Autodesk Fusion 360 part; units mm, degrees
(part 2 of 5)
  spline S301 degree 3 poles (-67.6031, -107.6158) (-67.9091, -107.753) (-68.2046, -107.8902) (-68.2574, -107.9113) knots 0 0 0 0 1 1 1 1
  spline S302 degree 3 poles (-68.2574, -107.9113) (-68.3629, -107.964) (-68.0041, -107.4364) (-67.5926, -106.9088) knots 0 0 0 0 1 1 1 1
  spline S303 degree 3 poles (-67.5926, -106.9088) (-67.276, -106.5289) (-67.1599, -106.4867) (-67.1599, -106.74) knots 0 0 0 0 1 1 1 1
  spline S304 degree 3 poles (-43.6395, -107.6791) (-43.4495, -107.9324) (-43.3229, -108.1434) (-43.344, -108.1434) knots 0 0 0 0 1 1 1 1
  spline S305 degree 3 poles (-43.344, -108.1434) (-43.3757, -108.1434) (-43.6078, -108.0273) (-43.8505, -107.8796) knots 0 0 0 0 1 1 1 1
  spline S306 degree 3 poles (-43.8505, -107.8796) (-44.1038, -107.7319) (-44.4098, -107.6158) (-44.5258, -107.6158) knots 0 0 0 0 1 1 1 1
  spline S307 degree 3 poles (-44.5258, -107.6158) (-44.9901, -107.6158) (-45.064, -107.2676) (-44.6947, -106.8772) knots 0 0 0 0 1 1 1 1
  spline S308 degree 3 poles (-44.6947, -106.8772) (-44.5364, -106.7083) (-44.5047, -106.7189) (-44.2515, -106.951) knots 0 0 0 0 1 1 1 1
  spline S309 degree 3 poles (-44.2515, -106.951) (-44.0932, -107.0988) (-43.8189, -107.4153) (-43.6395, -107.6791) knots 0 0 0 0 1 1 1 1
  spline S310 degree 3 poles (-45.3172, -106.9827) (-45.0323, -106.9827) (-45.0007, -107.0038) (-45.064, -107.2465) knots 0 0 0 0 1 1 1 1
  spline S311 degree 3 poles (-45.064, -107.2465) (-45.1062, -107.4364) (-45.0745, -107.5314) (-44.9585, -107.5736) knots 0 0 0 0 1 1 1 1
  spline S312 degree 3 poles (-44.9585, -107.5736) (-44.8424, -107.6158) (-44.8213, -107.6791) (-44.8952, -107.8057) knots 0 0 0 0 1 1 1 1
  spline S313 degree 3 poles (-44.8952, -107.8057) (-45.1695, -108.2911) (-45.1695, -108.2911) (-45.676, -107.9218) knots 0 0 0 0 1 1 1 1
  spline S314 degree 3 poles (-45.676, -107.9218) (-45.982, -107.7108) (-46.1508, -107.5208) (-46.1086, -107.4259) knots 0 0 0 0 1 1 1 1
  spline S315 degree 3 poles (-46.1086, -107.4259) (-46.077, -107.352) (-46.0559, -107.1621) (-46.0559, -107.0249) knots 0 0 0 0 1 1 1 1
  spline S316 degree 3 poles (-46.0559, -107.0249) (-46.0559, -106.8033) (-46.0242, -106.7822) (-45.8554, -106.8772) knots 0 0 0 0 1 1 1 1
  spline S317 degree 3 poles (-45.8554, -106.8772) (-45.7393, -106.9299) (-45.4966, -106.9827) (-45.3172, -106.9827) knots 0 0 0 0 1 1 1 1
  spline S318 degree 3 poles (-43.5234, -108.2173) (-42.2677, -108.9454) (-41.0542, -110.1166) (-40.5161, -111.1296) knots 0 0 0 0 1 1 1 1
  line L66 (-40.5161, -111.1296) -> (-40.2206, -111.6783)
  line L67 (-40.2206, -111.6783) -> (-40.6955, -111.2352)
  spline S319 degree 3 poles (-40.6955, -111.2352) (-41.4341, -110.5704) (-42.6792, -110.0006) (-43.6817, -109.8739) knots 0 0 0 0 1 1 1 1
  spline S320 degree 3 poles (-43.6817, -109.8739) (-44.2304, -109.8001) (-44.3042, -109.9161) (-43.7661, -110.0006) knots 0 0 0 0 1 1 1 1
  spline S321 degree 3 poles (-43.7661, -110.0006) (-42.8164, -110.1483) (-42.5632, -110.3804) (-42.1516, -111.4884) knots 0 0 0 0 1 1 1 1
  spline S322 degree 3 poles (-42.1516, -111.4884) (-41.8984, -112.1743) (-41.7295, -112.8918) (-41.8245, -112.8813) knots 0 0 0 0 1 1 1 1
  spline S323 degree 3 poles (-41.8245, -112.8813) (-41.8562, -112.8813) (-42.1516, -112.5647) (-42.4682, -112.1848) knots 0 0 0 0 1 1 1 1
  spline S324 degree 3 poles (-42.4682, -112.1848) (-43.0591, -111.4779) (-44.5153, -110.1905) (-45.2328, -109.7473) knots 0 0 0 0 1 1 1 1
  spline S325 degree 3 poles (-45.2328, -109.7473) (-45.581, -109.5363) (-45.6127, -109.473) (-45.5072, -109.3041) knots 0 0 0 0 1 1 1 1
  spline S326 degree 3 poles (-45.5072, -109.3041) (-45.4333, -109.1986) (-45.3489, -109.1247) (-45.3172, -109.1459) knots 0 0 0 0 1 1 1 1
  spline S327 degree 3 poles (-45.3172, -109.1459) (-45.2012, -109.2197) (-44.8846, -108.5655) (-44.9374, -108.3756) knots 0 0 0 0 1 1 1 1
  spline S328 degree 3 poles (-44.9374, -108.3756) (-44.9796, -108.2595) (-44.9163, -108.0906) (-44.7896, -107.9535) knots 0 0 0 0 1 1 1 1
  spline S329 degree 3 poles (-44.7896, -107.9535) (-44.5469, -107.7002) (-44.3676, -107.7319) (-43.5234, -108.2173) knots 0 0 0 0 1 1 1 1
  spline S330 degree 3 poles (-45.6866, -108.4283) (-45.6338, -108.6816) (-45.581, -108.7554) (-45.5494, -108.6394) knots 0 0 0 0 1 1 1 1
  spline S331 degree 3 poles (-45.5494, -108.6394) (-45.5283, -108.5233) (-45.4544, -108.4705) (-45.3594, -108.5022) knots 0 0 0 0 1 1 1 1
  spline S332 degree 3 poles (-45.3594, -108.5022) (-45.2645, -108.5338) (-45.2328, -108.5127) (-45.2645, -108.46) knots 0 0 0 0 1 1 1 1
  spline S333 degree 3 poles (-45.2645, -108.46) (-45.2961, -108.3967) (-45.275, -108.3544) (-45.2223, -108.3544) knots 0 0 0 0 1 1 1 1
  spline S334 degree 3 poles (-45.2223, -108.3544) (-45.064, -108.3544) (-45.0745, -108.7238) (-45.2328, -108.8609) knots 0 0 0 0 1 1 1 1
  spline S335 degree 3 poles (-45.2328, -108.8609) (-45.4333, -109.0192) (-46.0559, -108.7343) (-46.0559, -108.4916) knots 0 0 0 0 1 1 1 1
  spline S336 degree 3 poles (-46.0559, -108.4916) (-46.0559, -108.3861) (-46.0875, -108.1856) (-46.1297, -108.0484) knots 0 0 0 0 1 1 1 1
  spline S337 degree 3 poles (-46.1297, -108.0484) (-46.1825, -107.8268) (-46.172, -107.8163) (-45.982, -107.9218) knots 0 0 0 0 1 1 1 1
  spline S338 degree 3 poles (-45.982, -107.9218) (-45.8554, -107.9851) (-45.7288, -108.1962) (-45.6866, -108.4283) knots 0 0 0 0 1 1 1 1
  spline S339 degree 3 poles (-46.5096, -108.1645) (-46.5413, -108.2489) (-46.5729, -108.2173) (-46.5729, -108.1012) knots 0 0 0 0 1 1 1 1
  spline S340 degree 3 poles (-46.5729, -108.1012) (-46.5835, -107.9851) (-46.5518, -107.9218) (-46.5202, -107.964) knots 0 0 0 0 1 1 1 1
  spline S341 degree 3 poles (-46.5202, -107.964) (-46.4885, -107.9957) (-46.478, -108.0906) (-46.5096, -108.1645) knots 0 0 0 0 1 1 1 1
  line L68 (-45.8554, -108.9454) -> (-45.5177, -109.1142)
  line L69 (-45.5177, -109.1142) -> (-45.7604, -109.3991)
  spline S342 degree 3 poles (-45.7604, -109.3991) (-45.8976, -109.5468) (-46.0453, -109.7051) (-46.1086, -109.7473) knots 0 0 0 0 1 1 1 1
  spline S343 degree 3 poles (-46.1086, -109.7473) (-46.172, -109.8001) (-46.1192, -109.9056) (-45.9715, -110.0217) knots 0 0 0 0 1 1 1 1
  spline S344 degree 3 poles (-45.9715, -110.0217) (-45.7499, -110.1905) (-45.7499, -110.2116) (-45.9293, -110.3277) knots 0 0 0 0 1 1 1 1
  spline S345 degree 3 poles (-45.9293, -110.3277) (-46.1086, -110.4332) (-46.1614, -110.3804) (-46.4569, -109.8001) knots 0 0 0 0 1 1 1 1
  line L70 (-46.4569, -109.8001) -> (-46.7734, -109.1564)
  line L71 (-46.7734, -109.1564) -> (-46.4991, -108.977)
  spline S346 degree 3 poles (-46.4991, -108.977) (-46.3408, -108.8715) (-46.2142, -108.7871) (-46.2036, -108.7871) knots 0 0 0 0 1 1 1 1
  spline S347 degree 3 poles (-46.2036, -108.7871) (-46.2036, -108.7765) (-46.0453, -108.8504) (-45.8554, -108.9454) knots 0 0 0 0 1 1 1 1
  spline S348 degree 3 poles (-65.0073, -128.4877) (-65.1762, -129.0575) (-65.2606, -129.1314) (-65.4611, -128.8993) knots 0 0 0 0 1 1 1 1
  spline S349 degree 3 poles (-65.4611, -128.8993) (-65.5455, -128.7832) (-65.4927, -128.6566) (-65.2395, -128.3189) knots 0 0 0 0 1 1 1 1
  spline S350 degree 3 poles (-65.2395, -128.3189) (-65.0495, -128.0762) (-64.8913, -127.8968) (-64.8807, -127.9074) knots 0 0 0 0 1 1 1 1
  spline S351 degree 3 poles (-64.8807, -127.9074) (-64.8596, -127.9285) (-64.9229, -128.1817) (-65.0073, -128.4877) knots 0 0 0 0 1 1 1 1
  spline S352 degree 3 poles (-65.8409, -129.1947) (-65.8409, -129.3741) (-65.8831, -129.448) (-65.9781, -129.4057) knots 0 0 0 0 1 1 1 1
  spline S353 degree 3 poles (-65.9781, -129.4057) (-66.0625, -129.3741) (-66.1786, -129.353) (-66.2419, -129.353) knots 0 0 0 0 1 1 1 1
  spline S354 degree 3 poles (-66.2419, -129.353) (-66.3158, -129.353) (-66.2525, -129.258) (-66.1047, -129.1419) knots 0 0 0 0 1 1 1 1
  spline S355 degree 2 poles (-66.1047, -129.1419) (-65.957, -129.0259) (-65.8409, -128.9309) knots 0 0 0 1 1 1
  spline S356 degree 2 poles (-65.8409, -128.9309) (-65.8409, -129.047) (-65.8409, -129.1947) knots 0 0 0 1 1 1
  spline S357 degree 3 poles (-47.1638, -105.0939) (-47.2061, -105.1466) (-47.1638, -105.2838) (-47.0689, -105.3893) knots 0 0 0 0 1 1 1 1
  spline S358 degree 3 poles (-47.0689, -105.3893) (-46.9739, -105.4948) (-46.9211, -105.6004) (-46.9528, -105.632) knots 0 0 0 0 1 1 1 1
  spline S359 degree 3 poles (-46.9528, -105.632) (-46.9845, -105.6637) (-46.9211, -105.7164) (-46.7945, -105.7481) knots 0 0 0 0 1 1 1 1
  spline S360 degree 3 poles (-46.7945, -105.7481) (-46.5096, -105.822) (-46.5307, -105.6953) (-46.8578, -105.3893) knots 0 0 0 0 1 1 1 1
  line L72 (-46.8578, -105.3893) -> (-47.1322, -105.1361)
  line L73 (-47.1322, -105.1361) -> (-46.8262, -105.0728)
  line L74 (-46.8262, -105.0728) -> (-46.5307, -104.9989)
  line L75 (-46.5307, -104.9989) -> (-46.8156, -104.9884)
  spline S361 degree 3 poles (-46.8156, -104.9884) (-46.9739, -104.9884) (-47.1322, -105.0306) (-47.1638, -105.0939) knots 0 0 0 0 1 1 1 1
  spline S362 degree 3 poles (-47.0583, -105.9169) (-47.0056, -106.0225) (-47.1216, -106.0752) (-47.7125, -106.1913) knots 0 0 0 0 1 1 1 1
  spline S363 degree 3 poles (-47.7125, -106.1913) (-47.9025, -106.2335) (-48.0608, -106.2968) (-48.0608, -106.339) knots 0 0 0 0 1 1 1 1
  spline S364 degree 3 poles (-48.0608, -106.339) (-48.0608, -106.3812) (-47.7337, -106.3496) (-47.3327, -106.2546) knots 0 0 0 0 1 1 1 1
  spline S365 degree 3 poles (-47.3327, -106.2546) (-46.7101, -106.1174) (-46.6362, -106.0752) (-46.784, -105.9591) knots 0 0 0 0 1 1 1 1
  spline S366 degree 3 poles (-46.784, -105.9591) (-46.9845, -105.8009) (-47.1533, -105.7798) (-47.0583, -105.9169) knots 0 0 0 0 1 1 1 1
  spline S367 degree 3 poles (-48.0608, -106.8666) (-47.9447, -107.2992) (-47.8497, -107.4048) (-47.8497, -107.1304) knots 0 0 0 0 1 1 1 1
  spline S368 degree 3 poles (-47.8497, -107.1304) (-47.8497, -107.0143) (-47.9236, -106.8244) (-48.008, -106.7083) knots 0 0 0 0 1 1 1 1
  spline S369 degree 3 poles (-48.008, -106.7083) (-48.1452, -106.5289) (-48.1557, -106.5395) (-48.0608, -106.8666) knots 0 0 0 0 1 1 1 1
  spline S370 degree 3 poles (-64.8596, -105.1572) (-64.733, -105.1783) (-64.5219, -105.1783) (-64.3848, -105.1572) knots 0 0 0 0 1 1 1 1
  spline S371 degree 3 poles (-64.3848, -105.1572) (-64.2581, -105.1361) (-64.3637, -105.115) (-64.6275, -105.115) knots 0 0 0 0 1 1 1 1
  spline S372 degree 3 poles (-64.6275, -105.115) (-64.8913, -105.115) (-64.9968, -105.1361) (-64.8596, -105.1572) knots 0 0 0 0 1 1 1 1
  spline S373 degree 3 poles (-64.6063, -105.5054) (-65.0495, -105.7798) (-64.9546, -105.9275) (-64.3425, -105.9275) knots 0 0 0 0 1 1 1 1
  spline S374 degree 3 poles (-64.3425, -105.9275) (-63.8149, -105.9275) (-63.7622, -105.8642) (-64.2265, -105.8009) knots 0 0 0 0 1 1 1 1
  spline S375 degree 3 poles (-64.2265, -105.8009) (-64.6063, -105.7481) (-64.6908, -105.6426) (-64.427, -105.5582) knots 0 0 0 0 1 1 1 1
  spline S376 degree 3 poles (-64.427, -105.5582) (-64.3003, -105.5265) (-64.2054, -105.4421) (-64.2054, -105.3893) knots 0 0 0 0 1 1 1 1
  spline S377 degree 3 poles (-64.2054, -105.3893) (-64.2054, -105.2627) (-64.2054, -105.2627) (-64.6063, -105.5054) knots 0 0 0 0 1 1 1 1
  spline S378 degree 3 poles (-64.1315, -106.2229) (-64.3953, -106.5078) (-64.3531, -106.6661) (-64.0154, -106.6556) knots 0 0 0 0 1 1 1 1
  spline S379 degree 3 poles (-64.0154, -106.6556) (-63.7622, -106.6345) (-63.7516, -106.6345) (-63.9732, -106.5923) knots 0 0 0 0 1 1 1 1
  spline S380 degree 3 poles (-63.9732, -106.5923) (-64.2159, -106.5501) (-64.2159, -106.5395) (-64.0365, -106.339) knots 0 0 0 0 1 1 1 1
  spline S381 degree 3 poles (-64.0365, -106.339) (-63.9416, -106.2335) (-63.8783, -106.1174) (-63.9099, -106.0858) knots 0 0 0 0 1 1 1 1
  spline S382 degree 3 poles (-63.9099, -106.0858) (-63.9416, -106.0541) (-64.0365, -106.1174) (-64.1315, -106.2229) knots 0 0 0 0 1 1 1 1
  spline S383 degree 3 poles (-44.3465, -108.9454) (-44.663, -109.0298) (-45.0112, -109.167) (-45.1379, -109.2619) knots 0 0 0 0 1 1 1 1
  spline S384 degree 3 poles (-45.1379, -109.2619) (-45.3489, -109.4202) (-45.3489, -109.4308) (-45.159, -109.3569) knots 0 0 0 0 1 1 1 1
  spline S385 degree 3 poles (-45.159, -109.3569) (-44.6208, -109.167) (-44.262, -109.072) (-43.5762, -108.9348) knots 0 0 0 0 1 1 1 1
  spline S386 degree 3 poles (-43.5762, -108.9348) (-42.9008, -108.8082) (-42.8797, -108.7976) (-43.3124, -108.7976) knots 0 0 0 0 1 1 1 1
  spline S387 degree 3 poles (-43.3124, -108.7976) (-43.5762, -108.7871) (-44.0404, -108.8609) (-44.3465, -108.9454) knots 0 0 0 0 1 1 1 1
  spline S388 degree 3 poles (-45.2117, -109.5574) (-45.2117, -109.6101) (-44.5258, -109.9373) (-44.4098, -109.9373) knots 0 0 0 0 1 1 1 1
  spline S389 degree 3 poles (-44.4098, -109.9373) (-44.3887, -109.9373) (-44.3676, -109.895) (-44.3676, -109.8423) knots 0 0 0 0 1 1 1 1
  spline S390 degree 3 poles (-44.3676, -109.8423) (-44.3676, -109.7895) (-44.4836, -109.7157) (-44.6208, -109.684) knots 0 0 0 0 1 1 1 1
  spline S391 degree 3 poles (-44.6208, -109.684) (-44.758, -109.6523) (-44.9479, -109.589) (-45.0429, -109.5574) knots 0 0 0 0 1 1 1 1
  spline S392 degree 3 poles (-45.0429, -109.5574) (-45.1379, -109.5257) (-45.2117, -109.5257) (-45.2117, -109.5574) knots 0 0 0 0 1 1 1 1
  spline S393 degree 3 poles (-51.2791, -107.0038) (-50.5299, -107.9957) (-49.8546, -109.5679) (-49.4958, -111.098) knots 0 0 0 0 1 1 1 1
  spline S394 degree 3 poles (-49.4958, -111.098) (-49.1687, -112.5331) (-49.1476, -112.7019) (-49.0632, -114.2108) knots 0 0 0 0 1 1 1 1
  line L76 (-49.0632, -114.2108) -> (-48.9893, -115.3715)
  line L77 (-48.9893, -115.3715) -> (-49.2109, -115.1077)
  spline S395 degree 3 poles (-49.2109, -115.1077) (-50.1501, -113.9681) (-51.3741, -111.6256) (-51.3636, -110.9925) knots 0 0 0 0 1 1 1 1
  spline S396 degree 3 poles (-51.3636, -110.9925) (-51.3636, -110.7603) (-51.3847, -110.697) (-51.4269, -110.8131) knots 0 0 0 0 1 1 1 1
  spline S397 degree 3 poles (-51.4269, -110.8131) (-51.4796, -110.9502) (-51.5324, -110.8764) (-51.6379, -110.5176) knots 0 0 0 0 1 1 1 1
  spline S398 degree 3 poles (-51.6379, -110.5176) (-51.7118, -110.2538) (-51.8173, -110.0428) (-51.8595, -110.0428) knots 0 0 0 0 1 1 1 1
  spline S399 degree 3 poles (-51.8595, -110.0428) (-51.9545, -110.0428) (-51.8912, -110.296) (-51.6168, -111.0874) knots 0 0 0 0 1 1 1 1
  spline S400 degree 3 poles (-51.6168, -111.0874) (-51.5218, -111.3512) (-51.4691, -111.5939) (-51.5007, -111.6467) knots 0 0 0 0 1 1 1 1
  spline S401 degree 3 poles (-51.5007, -111.6467) (-51.5957, -111.7944) (-52.2921, -112.0477) (-52.4082, -111.9843) knots 0 0 0 0 1 1 1 1
  spline S402 degree 3 poles (-52.4082, -111.9843) (-52.5665, -111.8788) (-53.1891, -110.5071) (-53.3684, -109.8317) knots 0 0 0 0 1 1 1 1
  spline S403 degree 3 poles (-53.3684, -109.8317) (-53.4634, -109.5152) (-53.5584, -108.9137) (-53.59, -108.5127) knots 0 0 0 0 1 1 1 1
  spline S404 degree 3 poles (-53.59, -108.5127) (-53.6217, -108.1012) (-53.6956, -107.6264) (-53.7589, -107.4575) knots 0 0 0 0 1 1 1 1
  spline S405 degree 3 poles (-53.7589, -107.4575) (-53.8433, -107.1937) (-53.8538, -107.2359) (-53.8116, -107.7213) knots 0 0 0 0 1 1 1 1
  spline S406 degree 3 poles (-53.8116, -107.7213) (-53.6111, -110.1166) (-53.6428, -112.4697) (-53.8749, -112.4697) knots 0 0 0 0 1 1 1 1
  spline S407 degree 3 poles (-53.8749, -112.4697) (-53.9382, -112.4697) (-53.9488, -112.417) (-53.9066, -112.3431) knots 0 0 0 0 1 1 1 1
  spline S408 degree 3 poles (-53.9066, -112.3431) (-53.8538, -112.2693) (-53.8749, -112.2587) (-53.9594, -112.3009) knots 0 0 0 0 1 1 1 1
  spline S409 degree 3 poles (-53.9594, -112.3009) (-54.0649, -112.3642) (-54.0543, -112.4275) (-53.9488, -112.5542) knots 0 0 0 0 1 1 1 1
  spline S410 degree 3 poles (-53.9488, -112.5542) (-53.8222, -112.7019) (-53.8222, -112.8707) (-53.9277, -113.5249) knots 0 0 0 0 1 1 1 1
  line L78 (-53.9277, -113.5249) -> (-54.0438, -114.3163)
  line L79 (-54.0438, -114.3163) -> (-54.0649, -113.6832)
  spline S411 degree 3 poles (-54.0649, -113.6832) (-54.0754, -113.335) (-54.202, -112.3853) (-54.3498, -111.5728) knots 0 0 0 0 1 1 1 1
  spline S412 degree 3 poles (-54.3498, -111.5728) (-54.4975, -110.7603) (-54.6241, -109.6629) (-54.6347, -109.1247) knots 0 0 0 0 1 1 1 1
  spline S413 degree 3 poles (-54.6347, -109.1247) (-54.6663, -108.0906) (-54.7402, -107.8691) (-54.9829, -108.1856) knots 0 0 0 0 1 1 1 1
  spline S414 degree 3 poles (-54.9829, -108.1856) (-55.1834, -108.46) (-55.1728, -109.1353) (-54.9723, -109.3041) knots 0 0 0 0 1 1 1 1
  spline S415 degree 3 poles (-54.9723, -109.3041) (-54.793, -109.4519) (-54.7508, -109.3041) (-54.9196, -109.1353) knots 0 0 0 0 1 1 1 1
  spline S416 degree 3 poles (-54.9196, -109.1353) (-54.9829, -109.072) (-54.9934, -108.8715) (-54.9512, -108.6605) knots 0 0 0 0 1 1 1 1
  line L80 (-54.9512, -108.6605) -> (-54.8774, -108.3017)
  line L81 (-54.8774, -108.3017) -> (-54.8035, -108.7238)
  spline S417 degree 3 poles (-54.8035, -108.7238) (-54.6769, -109.3569) (-54.6874, -109.6418) (-54.8246, -109.5574) knots 0 0 0 0 1 1 1 1
  spline S418 degree 3 poles (-54.8246, -109.5574) (-54.8985, -109.5152) (-54.9196, -109.5574) (-54.8879, -109.684) knots 0 0 0 0 1 1 1 1
  spline S419 degree 3 poles (-54.8879, -109.684) (-54.6663, -110.4226) (-54.5925, -110.8342) (-54.392, -112.2587) knots 0 0 0 0 1 1 1 1
  spline S420 degree 3 poles (-54.392, -112.2587) (-54.2232, -113.4933) (-54.1176, -116.2052) (-54.1704, -117.7458) knots 0 0 0 0 1 1 1 1
  line L82 (-54.1704, -117.7458) -> (-54.1915, -118.3261)
  line L83 (-54.1915, -118.3261) -> (-54.5714, -117.904)
  spline S421 degree 3 poles (-54.5714, -117.904) (-55.3206, -117.0704) (-55.8693, -116.2263) (-55.8693, -115.9308) knots 0 0 0 0 1 1 1 1
  spline S422 degree 3 poles (-55.8693, -115.9308) (-55.8693, -115.3504) (-56.0592, -115.6459) (-56.1331, -116.3423) knots 0 0 0 0 1 1 1 1
  spline S423 degree 3 poles (-56.1331, -116.3423) (-56.228, -117.2709) (-56.3758, -117.6613) (-56.3863, -117.0177) knots 0 0 0 0 1 1 1 1
  spline S424 degree 3 poles (-56.3863, -117.0177) (-56.4074, -116.0152) (-57.4099, -112.4697) (-57.6737, -112.4697) knots 0 0 0 0 1 1 1 1
  spline S425 degree 3 poles (-57.6737, -112.4697) (-57.7264, -112.4697) (-57.6631, -112.7335) (-57.547, -113.0607) knots 0 0 0 0 1 1 1 1
  spline S426 degree 3 poles (-57.547, -113.0607) (-57.2832, -113.7676) (-56.6079, -116.0891) (-56.6501, -116.1313) knots 0 0 0 0 1 1 1 1
  spline S427 degree 3 poles (-56.6501, -116.1313) (-56.6712, -116.1524) (-56.8717, -115.8886) (-57.1039, -115.5615) knots 0 0 0 0 1 1 1 1
  spline S428 degree 3 poles (-57.1039, -115.5615) (-58.0746, -114.137) (-58.6128, -112.8918) (-58.3701, -112.5964) knots 0 0 0 0 1 1 1 1
  spline S429 degree 3 poles (-58.3701, -112.5964) (-58.2751, -112.4592) (-58.2751, -112.4486) (-58.3701, -112.5119) knots 0 0 0 0 1 1 1 1
  spline S430 degree 3 poles (-58.3701, -112.5119) (-58.444, -112.5542) (-58.5073, -112.5753) (-58.5178, -112.5542) knots 0 0 0 0 1 1 1 1
  spline S431 degree 3 poles (-58.5178, -112.5542) (-58.5178, -112.5331) (-58.5495, -112.3115) (-58.5811, -112.0477) knots 0 0 0 0 1 1 1 1
  spline S432 degree 3 poles (-58.5811, -112.0477) (-58.6656, -111.3723) (-58.7183, -111.3829) (-58.7183, -112.0899) knots 0 0 0 0 1 1 1 1
  spline S433 degree 3 poles (-58.7183, -112.0899) (-58.7183, -112.6808) (-58.7289, -112.7019) (-58.9505, -112.6386) knots 0 0 0 0 1 1 1 1
  spline S434 degree 3 poles (-58.9505, -112.6386) (-59.0876, -112.6069) (-59.267, -112.5753) (-59.3514, -112.5647) knots 0 0 0 0 1 1 1 1
  spline S435 degree 3 poles (-59.3514, -112.5647) (-59.4359, -112.5542) (-59.3409, -112.5119) (-59.1404, -112.4697) knots 0 0 0 0 1 1 1 1
  line L84 (-59.1404, -112.4697) -> (-58.7711, -112.3959)
  line L85 (-58.7711, -112.3959) -> (-59.0982, -112.3748)
  spline S436 degree 3 poles (-59.0982, -112.3748) (-59.5097, -112.3642) (-59.5519, -112.2376) (-59.6363, -110.7814) knots 0 0 0 0 1 1 1 1
  spline S437 degree 3 poles (-59.6363, -110.7814) (-59.6997, -109.5996) (-59.5414, -108.5127) (-59.1298, -107.3309) knots 0 0 0 0 1 1 1 1
  spline S438 degree 3 poles (-59.1298, -107.3309) (-58.9083, -106.6872) (-58.8766, -106.4129) (-59.0349, -106.6661) knots 0 0 0 0 1 1 1 1
  spline S439 degree 3 poles (-59.0349, -106.6661) (-59.2459, -106.9827) (-59.5625, -108.1223) (-59.7735, -109.2197) knots 0 0 0 0 1 1 1 1
  spline S440 degree 3 poles (-59.7735, -109.2197) (-59.974, -110.3171) (-60.6177, -111.9421) (-60.8604, -111.9421) knots 0 0 0 0 1 1 1 1
  spline S441 degree 3 poles (-60.8604, -111.9421) (-60.9131, -111.9421) (-61.0925, -111.8472) (-61.2614, -111.7205) knots 0 0 0 0 1 1 1 1
  spline S442 degree 3 poles (-61.2614, -111.7205) (-61.4302, -111.6045) (-61.5674, -111.5517) (-61.5674, -111.615) knots 0 0 0 0 1 1 1 1
  spline S443 degree 3 poles (-61.5674, -111.615) (-61.5674, -111.6783) (-61.5357, -111.7311) (-61.4829, -111.7311) knots 0 0 0 0 1 1 1 1
  spline S444 degree 3 poles (-61.4829, -111.7311) (-61.4407, -111.7417) (-61.3036, -111.8261) (-61.1664, -111.9421) knots 0 0 0 0 1 1 1 1
  line L86 (-61.1664, -111.9421) -> (-60.9237, -112.1426)
  line L87 (-60.9237, -112.1426) -> (-61.4829, -113.124)
  spline S445 degree 3 poles (-61.4829, -113.124) (-61.7995, -113.6621) (-62.1794, -114.3902) (-62.3377, -114.7384) knots 0 0 0 0 1 1 1 1
  line L88 (-62.3377, -114.7384) -> (-62.6331, -115.3715)
  line L89 (-62.6331, -115.3715) -> (-62.5804, -114.8756)
  spline S446 degree 3 poles (-62.5804, -114.8756) (-62.5276, -114.3586) (-61.9261, -111.921) (-61.7573, -111.5728) knots 0 0 0 0 1 1 1 1
  spline S447 degree 3 poles (-61.7573, -111.5728) (-61.6623, -111.3723) (-61.6623, -111.3618) (-61.8206, -111.5623) knots 0 0 0 0 1 1 1 1
  spline S448 degree 3 poles (-61.8206, -111.5623) (-61.9789, -111.7628) (-62.1266, -112.2059) (-62.5382, -113.736) knots 0 0 0 0 1 1 1 1
  spline S449 degree 3 poles (-62.5382, -113.736) (-62.8231, -114.7912) (-62.918, -117.4397) (-62.6964, -118.2417) knots 0 0 0 0 1 1 1 1
  spline S450 degree 3 poles (-62.6964, -118.2417) (-62.517, -118.917) (-62.6437, -118.8854) (-62.8653, -118.1995) knots 0 0 0 0 1 1 1 1
  spline S451 degree 3 poles (-62.8653, -118.1995) (-63.3084, -116.8383) (-63.3929, -116.2896) (-63.414, -114.8545) knots 0 0 0 0 1 1 1 1
  spline S452 degree 3 poles (-63.414, -114.8545) (-63.4245, -113.9892) (-63.4773, -113.3667) (-63.5406, -113.3456) knots 0 0 0 0 1 1 1 1
  spline S453 degree 3 poles (-63.5406, -113.3456) (-63.6567, -113.3034) (-63.6461, -115.6142) (-63.5195, -116.374) knots 0 0 0 0 1 1 1 1
  spline S454 degree 3 poles (-63.5195, -116.374) (-63.1924, -118.4105) (-62.0844, -120.4471) (-60.9026, -121.1963) knots 0 0 0 0 1 1 1 1
  spline S455 degree 3 poles (-60.9026, -121.1963) (-60.681, -121.3334) (-60.5122, -121.4706) (-60.5333, -121.5023) knots 0 0 0 0 1 1 1 1
  spline S456 degree 3 poles (-60.5333, -121.5023) (-60.6493, -121.6078) (-61.7679, -121.3018) (-62.401, -120.9958) knots 0 0 0 0 1 1 1 1
  spline S457 degree 3 poles (-62.401, -120.9958) (-63.1713, -120.6265) (-64.3848, -119.5079) (-64.638, -118.9276) knots 0 0 0 0 1 1 1 1
  spline S458 degree 3 poles (-64.638, -118.9276) (-64.7752, -118.611) (-64.944, -118.4738) (-64.944, -118.6743) knots 0 0 0 0 1 1 1 1
  spline S459 degree 3 poles (-64.944, -118.6743) (-64.944, -118.8537) (-64.0682, -120.025) (-63.5828, -120.4893) knots 0 0 0 0 1 1 1 1
  spline S460 degree 3 poles (-63.5828, -120.4893) (-63.319, -120.7531) (-62.8864, -121.344) (-62.6331, -121.7977) knots 0 0 0 0 1 1 1 1
  spline S461 degree 3 poles (-62.6331, -121.7977) (-62.3799, -122.2409) (-62.1055, -122.6419) (-62.0317, -122.6736) knots 0 0 0 0 1 1 1 1
  spline S462 degree 3 poles (-62.0317, -122.6736) (-61.9472, -122.7052) (-61.8839, -122.7896) (-61.8839, -122.8635) knots 0 0 0 0 1 1 1 1
  spline S463 degree 3 poles (-61.8839, -122.8635) (-61.8839, -122.9374) (-61.8101, -123.0218) (-61.7256, -123.064) knots 0 0 0 0 1 1 1 1
  spline S464 degree 3 poles (-61.7256, -123.064) (-61.6412, -123.0956) (-61.5674, -123.0851) (-61.5674, -123.0323) knots 0 0 0 0 1 1 1 1
  spline S465 degree 3 poles (-61.5674, -123.0323) (-61.5674, -122.9796) (-61.293, -123.0534) (-60.9553, -123.1906) knots 0 0 0 0 1 1 1 1
  spline S466 degree 3 poles (-60.9553, -123.1906) (-60.5438, -123.3489) (-60.3433, -123.4966) (-60.3222, -123.6443) knots 0 0 0 0 1 1 1 1
  spline S467 degree 3 poles (-60.3222, -123.6443) (-60.28, -123.9081) (-60.6599, -125.5332) (-60.892, -126.0502) knots 0 0 0 0 1 1 1 1
  line L90 (-60.892, -126.0502) -> (-61.0714, -126.4512)
  line L91 (-61.0714, -126.4512) -> (-61.2191, -125.5543)
  spline S468 degree 3 poles (-61.2191, -125.5543) (-61.3036, -125.0689) (-61.4935, -124.3513) (-61.6412, -123.9715) knots 0 0 0 0 1 1 1 1
  spline S469 degree 3 poles (-61.6412, -123.9715) (-61.7784, -123.5916) (-61.9261, -123.1801) (-61.9578, -123.064) knots 0 0 0 0 1 1 1 1
  spline S470 degree 3 poles (-61.9578, -123.064) (-61.9894, -122.9374) (-62.1794, -122.7474) (-62.3904, -122.6419) knots 0 0 0 0 1 1 1 1
  spline S471 degree 3 poles (-62.3904, -122.6419) (-63.0024, -122.3253) (-63.6883, -121.8505) (-64.1737, -121.4073) knots 0 0 0 0 1 1 1 1
  spline S472 degree 3 poles (-64.1737, -121.4073) (-64.427, -121.1752) (-64.6275, -121.038) (-64.6275, -121.0907) knots 0 0 0 0 1 1 1 1
  spline S473 degree 3 poles (-64.6275, -121.0907) (-64.6275, -121.344) (-62.6753, -122.8107) (-62.3377, -122.8107) knots 0 0 0 0 1 1 1 1
  spline S474 degree 3 poles (-62.3377, -122.8107) (-62.2638, -122.8107) (-62.2005, -122.8846) (-62.2005, -122.9796) knots 0 0 0 0 1 1 1 1
  spline S475 degree 3 poles (-62.2005, -122.9796) (-62.2005, -123.1273) (-62.2216, -123.1378) (-62.3799, -123.0112) knots 0 0 0 0 1 1 1 1
  spline S476 degree 3 poles (-62.3799, -123.0112) (-62.5487, -122.874) (-62.5593, -122.8846) (-62.4221, -123.0429) knots 0 0 0 0 1 1 1 1
  spline S477 degree 3 poles (-62.4221, -123.0429) (-62.3482, -123.1484) (-62.2427, -123.2117) (-62.2005, -123.1801) knots 0 0 0 0 1 1 1 1
  spline S478 degree 3 poles (-62.2005, -123.1801) (-62.1477, -123.1484) (-62.0105, -123.4016) (-61.8839, -123.7288) knots 0 0 0 0 1 1 1 1
  spline S479 degree 3 poles (-61.8839, -123.7288) (-61.6096, -124.4674) (-61.1242, -126.6306) (-61.2614, -126.5461) knots 0 0 0 0 1 1 1 1
  spline S480 degree 3 poles (-61.2614, -126.5461) (-61.3141, -126.5145) (-61.3563, -126.4406) (-61.3563, -126.3879) knots 0 0 0 0 1 1 1 1
  spline S481 degree 3 poles (-61.3563, -126.3879) (-61.3563, -126.219) (-61.6729, -125.5226) (-61.7256, -125.5754) knots 0 0 0 0 1 1 1 1
  spline S482 degree 3 poles (-61.7256, -125.5754) (-61.7573, -125.5965) (-61.6518, -125.9341) (-61.5041, -126.3035) knots 0 0 0 0 1 1 1 1
  spline S483 degree 3 poles (-61.5041, -126.3035) (-60.9026, -127.7702) (-60.681, -129.7962) (-60.9448, -131.4634) knots 0 0 0 0 1 1 1 1
  spline S484 degree 3 poles (-60.9448, -131.4634) (-61.0503, -132.1598) (-61.0398, -132.2126) (-60.7865, -132.6558) knots 0 0 0 0 1 1 1 1
  spline S485 degree 3 poles (-60.7865, -132.6558) (-60.6388, -132.909) (-60.5122, -133.215) (-60.5122, -133.3417) knots 0 0 0 0 1 1 1 1
  spline S486 degree 3 poles (-60.5122, -133.3417) (-60.5122, -133.5632) (-60.3222, -134.1225) (-60.0268, -134.8084) knots 0 0 0 0 1 1 1 1
  spline S487 degree 3 poles (-60.0268, -134.8084) (-59.8157, -135.2727) (-59.8474, -135.4626) (-60.1112, -135.5154) knots 0 0 0 0 1 1 1 1
  spline S488 degree 3 poles (-60.1112, -135.5154) (-60.7338, -135.6314) (-60.9237, -135.5576) (-61.0714, -135.1355) knots 0 0 0 0 1 1 1 1
  spline S489 degree 3 poles (-61.0714, -135.1355) (-61.1136, -134.9983) (-61.0925, -134.9667) (-60.9553, -135.0089) knots 0 0 0 0 1 1 1 1
  spline S490 degree 3 poles (-60.9553, -135.0089) (-60.7865, -135.0616) (-60.7865, -135.0616) (-60.9553, -134.9561) knots 0 0 0 0 1 1 1 1
  spline S491 degree 3 poles (-60.9553, -134.9561) (-61.2297, -134.7767) (-61.8839, -133.7954) (-62.0528, -133.3311) knots 0 0 0 0 1 1 1 1
  spline S492 degree 3 poles (-62.0528, -133.3311) (-62.1372, -133.0884) (-62.1899, -132.7085) (-62.1583, -132.4658) knots 0 0 0 0 1 1 1 1
  spline S493 degree 3 poles (-62.1583, -132.4658) (-62.1372, -132.2337) (-62.1055, -131.9171) (-62.1055, -131.7694) knots 0 0 0 0 1 1 1 1
  spline S494 degree 3 poles (-62.1055, -131.7694) (-62.095, -131.6217) (-61.9789, -131.3579) (-61.8312, -131.189) knots 0 0 0 0 1 1 1 1
  spline S495 degree 3 poles (-61.8312, -131.189) (-61.4935, -130.7986) (-61.3247, -130.9569) (-61.3141, -131.6639) knots 0 0 0 0 1 1 1 1
  spline S496 degree 3 poles (-61.3141, -131.6639) (-61.3036, -131.9488) (-61.2614, -132.1598) (-61.2086, -132.1282) knots 0 0 0 0 1 1 1 1
  spline S497 degree 3 poles (-61.2086, -132.1282) (-61.0609, -132.0332) (-61.2508, -130.2394) (-61.4513, -129.7751) knots 0 0 0 0 1 1 1 1
  spline S498 degree 3 poles (-61.4513, -129.7751) (-61.5674, -129.5113) (-61.5674, -129.5113) (-61.5252, -129.8278) knots 0 0 0 0 1 1 1 1
  spline S499 degree 3 poles (-61.5252, -129.8278) (-61.4091, -130.6403) (-62.7281, -132.1071) (-63.9205, -132.4975) knots 0 0 0 0 1 1 1 1
  spline S500 degree 3 poles (-63.9205, -132.4975) (-64.8701, -132.8035) (-65.3344, -132.7507) (-66.4741, -132.2126) knots 0 0 0 0 1 1 1 1
  spline S501 degree 3 poles (-66.4741, -132.2126) (-66.5268, -132.1915) (-66.5163, -132.2442) (-66.4318, -132.3498) knots 0 0 0 0 1 1 1 1
  spline S502 degree 3 poles (-66.4318, -132.3498) (-66.0414, -132.8141) (-64.9651, -133.0145) (-64.121, -132.7718) knots 0 0 0 0 1 1 1 1
  spline S503 degree 3 poles (-64.121, -132.7718) (-63.5089, -132.5925) (-62.6437, -132.086) (-62.4854, -131.8222) knots 0 0 0 0 1 1 1 1
  spline S504 degree 3 poles (-62.4854, -131.8222) (-62.3271, -131.5478) (-62.211, -131.6744) (-62.3271, -132.0015) knots 0 0 0 0 1 1 1 1
  spline S505 degree 3 poles (-62.3271, -132.0015) (-62.4326, -132.3181) (-62.401, -133.0356) (-62.2532, -133.3944) knots 0 0 0 0 1 1 1 1
  spline S506 degree 3 poles (-62.2532, -133.3944) (-62.1794, -133.5738) (-62.2005, -133.5632) (-62.5276, -133.3839) knots 0 0 0 0 1 1 1 1
  spline S507 degree 3 poles (-62.5276, -133.3839) (-62.9708, -133.1306) (-63.4351, -133.0145) (-63.5089, -133.1306) knots 0 0 0 0 1 1 1 1
  spline S508 degree 3 poles (-63.5089, -133.1306) (-63.5406, -133.1834) (-63.2873, -133.2994) (-62.9391, -133.3944) knots 0 0 0 0 1 1 1 1
  spline S509 degree 3 poles (-62.9391, -133.3944) (-62.4432, -133.5421) (-62.2638, -133.6477) (-62.0317, -133.9642) knots 0 0 0 0 1 1 1 1
  spline S510 degree 3 poles (-62.0317, -133.9642) (-61.8734, -134.1858) (-61.6307, -134.4813) (-61.5041, -134.629) knots 0 0 0 0 1 1 1 1
  spline S511 degree 3 poles (-61.5041, -134.629) (-61.293, -134.8611) (-61.0714, -135.5048) (-61.1242, -135.7053) knots 0 0 0 0 1 1 1 1
  spline S512 degree 3 poles (-61.1242, -135.7053) (-61.1347, -135.7581) (-60.8182, -135.7897) (-60.4066, -135.7897) knots 0 0 0 0 1 1 1 1
  line L92 (-60.4066, -135.7897) -> (-59.668, -135.7897)
  line L93 (-59.668, -135.7897) -> (-59.668, -135.431)
  spline S513 degree 3 poles (-59.668, -135.431) (-59.668, -135.241) (-59.7841, -134.8084) (-59.9424, -134.4918) knots 0 0 0 0 1 1 1 1
  spline S514 degree 3 poles (-59.9424, -134.4918) (-60.0901, -134.1647) (-60.2378, -133.6688) (-60.2906, -133.3944) knots 0 0 0 0 1 1 1 1
  spline S515 degree 3 poles (-60.2906, -133.3944) (-60.3961, -132.698) (-60.2378, -130.9569) (-60.0057, -130.2288) knots 0 0 0 0 1 1 1 1
  spline S516 degree 3 poles (-60.0057, -130.2288) (-59.8368, -129.7012) (-59.763, -129.6168) (-59.5308, -129.5851) knots 0 0 0 0 1 1 1 1
  spline S517 degree 3 poles (-59.5308, -129.5851) (-59.2037, -129.5429) (-59.1932, -129.5746) (-59.3936, -130.1444) knots 0 0 0 0 1 1 1 1
  spline S518 degree 3 poles (-59.3936, -130.1444) (-59.4781, -130.3765) (-59.5941, -130.9358) (-59.6574, -131.379) knots 0 0 0 0 1 1 1 1
  spline S519 degree 3 poles (-59.6574, -131.379) (-59.7946, -132.3392) (-59.6258, -133.4999) (-59.2459, -134.3969) knots 0 0 0 0 1 1 1 1
  spline S520 degree 3 poles (-59.2459, -134.3969) (-59.0665, -134.8084) (-59.0243, -135.0511) (-59.0771, -135.3676) knots 0 0 0 0 1 1 1 1
  line L94 (-59.0771, -135.3676) -> (-59.1404, -135.7897)
  line L95 (-59.1404, -135.7897) -> (-56.0803, -135.7897)
  line L96 (-56.0803, -135.7897) -> (-53.0202, -135.7897)
  line L97 (-53.0202, -135.7897) -> (-53.0202, -135.3149)
  spline S521 degree 3 poles (-53.0202, -135.3149) (-53.0202, -135.0511) (-52.9569, -134.6712) (-52.8725, -134.4813) knots 0 0 0 0 1 1 1 1
  spline S522 degree 3 poles (-52.8725, -134.4813) (-52.5665, -133.7321) (-52.461, -132.4869) (-52.6087, -131.3051) knots 0 0 0 0 1 1 1 1
  spline S523 degree 3 poles (-52.6087, -131.3051) (-52.7775, -130.0494) (-53.1152, -128.4033) (-53.2946, -127.9918) knots 0 0 0 0 1 1 1 1
  spline S524 degree 3 poles (-53.2946, -127.9918) (-53.4212, -127.6963) (-53.4317, -127.6119) (-53.3157, -127.5486) knots 0 0 0 0 1 1 1 1
  spline S525 degree 3 poles (-53.3157, -127.5486) (-53.2313, -127.4958) (-53.1574, -127.538) (-53.1046, -127.6647) knots 0 0 0 0 1 1 1 1
  spline S526 degree 3 poles (-53.1046, -127.6647) (-53.0624, -127.7807) (-52.978, -127.8757) (-52.9147, -127.8757) knots 0 0 0 0 1 1 1 1
  spline S527 degree 3 poles (-52.9147, -127.8757) (-52.8619, -127.8757) (-52.8092, -127.9601) (-52.8092, -128.0656) knots 0 0 0 0 1 1 1 1
  spline S528 degree 3 poles (-52.8092, -128.0656) (-52.8092, -128.1712) (-52.7564, -128.3083) (-52.6931, -128.3716) knots 0 0 0 0 1 1 1 1
  spline S529 degree 3 poles (-52.6931, -128.3716) (-52.5981, -128.4666) (-52.2921, -129.7223) (-52.0705, -130.9358) knots 0 0 0 0 1 1 1 1
  spline S530 degree 3 poles (-52.0705, -130.9358) (-51.9123, -131.7483) (-52.0178, -133.3417) (-52.271, -134.0697) knots 0 0 0 0 1 1 1 1
  spline S531 degree 3 poles (-52.271, -134.0697) (-52.3871, -134.4285) (-52.4926, -134.9667) (-52.4926, -135.2621) knots 0 0 0 0 1 1 1 1
  line L98 (-52.4926, -135.2621) -> (-52.4926, -135.7897)
  line L99 (-52.4926, -135.7897) -> (-52.1233, -135.7897)
  spline S532 degree 3 poles (-52.1233, -135.7897) (-51.754, -135.7897) (-51.754, -135.7897) (-51.754, -135.3254) knots 0 0 0 0 1 1 1 1
  spline S533 degree 3 poles (-51.754, -135.3254) (-51.754, -135.0722) (-51.6801, -134.6818) (-51.5851, -134.4602) knots 0 0 0 0 1 1 1 1
  spline S534 degree 3 poles (-51.5851, -134.4602) (-51.2369, -133.6266) (-51.1314, -132.4658) (-51.2897, -130.9886) knots 0 0 0 0 1 1 1 1
  spline S535 degree 3 poles (-51.2897, -130.9886) (-51.4269, -129.7434) (-51.6907, -128.1606) (-51.8489, -127.7491) knots 0 0 0 0 1 1 1 1
  spline S536 degree 3 poles (-51.8489, -127.7491) (-51.8912, -127.6225) (-51.965, -127.2953) (-51.9967, -127.0315) knots 0 0 0 0 1 1 1 1
  spline S537 degree 3 poles (-51.9967, -127.0315) (-52.06, -126.6306) (-52.0283, -126.5145) (-51.8067, -126.2401) knots 0 0 0 0 1 1 1 1
  line L100 (-51.8067, -126.2401) -> (-51.5429, -125.9236)
  line L101 (-51.5429, -125.9236) -> (-51.5429, -126.3984)
  spline S538 degree 3 poles (-51.5429, -126.3984) (-51.5324, -126.6622) (-51.4902, -127.0632) (-51.4374, -127.2953) knots 0 0 0 0 1 1 1 1
  spline S539 degree 3 poles (-51.4374, -127.2953) (-50.8043, -130.1444) (-50.6777, -130.9252) (-50.6882, -132.0965) knots 0 0 0 0 1 1 1 1
  spline S540 degree 3 poles (-50.6882, -132.0965) (-50.6882, -133.0462) (-50.741, -133.4577) (-50.9204, -133.9959) knots 0 0 0 0 1 1 1 1
  spline S541 degree 3 poles (-50.9204, -133.9959) (-51.047, -134.3758) (-51.1736, -134.935) (-51.2158, -135.2305) knots 0 0 0 0 1 1 1 1
  line L102 (-51.2158, -135.2305) -> (-51.2897, -135.7897)
  line L103 (-51.2897, -135.7897) -> (-50.836, -135.7897)
  spline S542 degree 3 poles (-50.836, -135.7897) (-50.4033, -135.7897) (-50.3822, -135.7686) (-50.3822, -135.4837) knots 0 0 0 0 1 1 1 1
  spline S543 degree 3 poles (-50.3822, -135.4837) (-50.3822, -135.241) (-50.3295, -135.1672) (-50.1184, -135.1355) knots 0 0 0 0 1 1 1 1
  spline S544 degree 3 poles (-50.1184, -135.1355) (-49.9285, -135.0933) (-49.8546, -135.1249) (-49.8546, -135.2516) knots 0 0 0 0 1 1 1 1
  spline S545 degree 3 poles (-49.8546, -135.2516) (-49.8546, -135.4732) (-49.9707, -135.642) (-50.1712, -135.7159) knots 0 0 0 0 1 1 1 1
  spline S546 degree 3 poles (-50.1712, -135.7159) (-50.2767, -135.7581) (-50.2556, -135.7792) (-50.0973, -135.7792) knots 0 0 0 0 1 1 1 1
  spline S547 degree 3 poles (-50.0973, -135.7792) (-49.9074, -135.7897) (-49.8335, -135.6948) (-49.728, -135.3465) knots 0 0 0 0 1 1 1 1
  spline S548 degree 3 poles (-49.728, -135.3465) (-49.6647, -135.0933) (-49.4431, -134.6818) (-49.2531, -134.4285) knots 0 0 0 0 1 1 1 1
  spline S549 degree 3 poles (-49.2531, -134.4285) (-49.0632, -134.1753) (-48.9049, -133.922) (-48.9049, -133.8798) knots 0 0 0 0 1 1 1 1
  spline S550 degree 3 poles (-48.9049, -133.8798) (-48.9049, -133.7321) (-48.0819, -133.3522) (-47.7125, -133.3417) knots 0 0 0 0 1 1 1 1
  spline S551 degree 3 poles (-47.7125, -133.3417) (-47.5332, -133.3311) (-47.1638, -133.3311) (-46.9106, -133.3417) knots 0 0 0 0 1 1 1 1
  line L104 (-46.9106, -133.3417) -> (-46.4463, -133.3628)
  line L105 (-46.4463, -133.3628) -> (-46.6468, -133.5844)
  line L106 (-46.6468, -133.5844) -> (-46.8473, -133.8059)
  line L107 (-46.8473, -133.8059) -> (-46.4674, -133.616)
  spline S552 degree 3 poles (-46.4674, -133.616) (-46.0242, -133.3839) (-46.0242, -133.3417) (-46.4991, -133.2889) knots 0 0 0 0 1 1 1 1
  spline S553 degree 3 poles (-46.4991, -133.2889) (-46.689, -133.2678) (-46.9423, -133.2361) (-47.0583, -133.215) knots 0 0 0 0 1 1 1 1
  spline S554 degree 3 poles (-47.0583, -133.215) (-47.1849, -133.2045) (-47.3327, -133.1623) (-47.3854, -133.1201) knots 0 0 0 0 1 1 1 1
  spline S555 degree 3 poles (-47.3854, -133.1201) (-47.5332, -133.0356) (-48.2296, -133.2256) (-48.5567, -133.4366) knots 0 0 0 0 1 1 1 1
  spline S556 degree 3 poles (-48.5567, -133.4366) (-48.7994, -133.5949) (-48.8944, -133.4999) (-48.6833, -133.2889) knots 0 0 0 0 1 1 1 1
  spline S557 degree 3 poles (-48.6833, -133.2889) (-48.4723, -133.0779) (-48.5567, -131.9488) (-48.8311, -131.2418) knots 0 0 0 0 1 1 1 1
  spline S558 degree 3 poles (-48.8311, -131.2418) (-48.9788, -130.8725) (-49.116, -130.4293) (-49.1476, -130.2499) knots 0 0 0 0 1 1 1 1
  spline S559 degree 3 poles (-49.1476, -130.2499) (-49.2004, -129.9545) (-49.1898, -129.9545) (-49.0527, -130.1444) knots 0 0 0 0 1 1 1 1
  spline S560 degree 3 poles (-49.0527, -130.1444) (-48.2929, -131.2312) (-46.9423, -131.991) (-45.771, -131.991) knots 0 0 0 0 1 1 1 1
  spline S561 degree 3 poles (-45.771, -131.991) (-45.0323, -131.991) (-43.84, -131.4528) (-43.84, -131.1152) knots 0 0 0 0 1 1 1 1
  spline S562 degree 3 poles (-43.84, -131.1152) (-43.84, -131.0519) (-43.8927, -131.0519) (-43.9666, -131.1257) knots 0 0 0 0 1 1 1 1
  spline S563 degree 3 poles (-43.9666, -131.1257) (-44.0615, -131.189) (-44.2726, -131.1785) (-44.6314, -131.0835) knots 0 0 0 0 1 1 1 1
  spline S564 degree 3 poles (-44.6314, -131.0835) (-44.9163, -131.0097) (-45.1906, -130.9463) (-45.2328, -130.9358) knots 0 0 0 0 1 1 1 1
  spline S565 degree 3 poles (-45.2328, -130.9358) (-45.275, -130.9358) (-45.3278, -130.8408) (-45.37, -130.7248) knots 0 0 0 0 1 1 1 1
  spline S566 degree 3 poles (-45.37, -130.7248) (-45.4017, -130.6087) (-45.5916, -130.2816) (-45.7921, -129.9967) knots 0 0 0 0 1 1 1 1
  spline S567 degree 3 poles (-45.7921, -129.9967) (-46.0875, -129.5746) (-46.1192, -129.4691) (-45.9926, -129.4163) knots 0 0 0 0 1 1 1 1
  spline S568 degree 3 poles (-45.9926, -129.4163) (-45.6127, -129.2686) (-45.4966, -129.3424) (-45.5705, -129.6907) knots 0 0 0 0 1 1 1 1
  spline S569 degree 3 poles (-45.5705, -129.6907) (-45.6338, -130.0072) (-45.6232, -130.0178) (-45.4333, -129.8384) knots 0 0 0 0 1 1 1 1
  spline S570 degree 3 poles (-45.4333, -129.8384) (-45.1801, -129.6062) (-44.2198, -129.4585) (-43.7872, -129.5746) knots 0 0 0 0 1 1 1 1
  spline S571 degree 3 poles (-43.7872, -129.5746) (-43.5973, -129.6273) (-43.3124, -129.7751) (-43.1646, -129.8911) knots 0 0 0 0 1 1 1 1
  spline S572 degree 3 poles (-43.1646, -129.8911) (-42.9114, -130.0916) (-42.8375, -130.1022) (-42.3521, -129.9967) knots 0 0 0 0 1 1 1 1
  spline S573 degree 3 poles (-42.3521, -129.9967) (-42.0672, -129.9333) (-41.7929, -129.8806) (-41.7612, -129.8806) knots 0 0 0 0 1 1 1 1
  spline S574 degree 3 poles (-41.7612, -129.8806) (-41.6346, -129.8806) (-42.3943, -130.5137) (-42.5948, -130.577) knots 0 0 0 0 1 1 1 1
  spline S575 degree 3 poles (-42.5948, -130.577) (-42.7003, -130.6087) (-42.7848, -130.6825) (-42.7848, -130.7353) knots 0 0 0 0 1 1 1 1
  spline S576 degree 3 poles (-42.7848, -130.7353) (-42.7848, -130.8619) (-42.7214, -130.8514) (-42.3732, -130.672) knots 0 0 0 0 1 1 1 1
  spline S577 degree 3 poles (-42.3732, -130.672) (-42.0989, -130.5348) (-42.0145, -130.5348) (-41.5607, -130.6931) knots 0 0 0 0 1 1 1 1
  spline S578 degree 3 poles (-41.5607, -130.6931) (-41.2653, -130.7881) (-40.8537, -131.0624) (-40.5477, -131.3579) knots 0 0 0 0 1 1 1 1
  spline S579 degree 3 poles (-40.5477, -131.3579) (-40.0412, -131.8433) (-39.8513, -131.8327) (-40.2523, -131.3262) knots 0 0 0 0 1 1 1 1
  spline S580 degree 3 poles (-40.2523, -131.3262) (-40.495, -131.0202) (-41.2336, -130.5665) (-41.6662, -130.4504) knots 0 0 0 0 1 1 1 1
  spline S581 degree 3 poles (-41.6662, -130.4504) (-41.9511, -130.3871) (-41.9511, -130.3765) (-41.7612, -130.1866) knots 0 0 0 0 1 1 1 1
  spline S582 degree 3 poles (-41.7612, -130.1866) (-41.5185, -129.9333) (-41.0542, -129.9122) (-40.4844, -130.1233) knots 0 0 0 0 1 1 1 1
  spline S583 degree 3 poles (-40.4844, -130.1233) (-39.7458, -130.3976) (-39.9463, -130.0811) (-40.7588, -129.7012) knots 0 0 0 0 1 1 1 1
  spline S584 degree 3 poles (-40.7588, -129.7012) (-42.0567, -129.0786) (-43.0697, -127.8546) (-44.2093, -125.5015) knots 0 0 0 0 1 1 1 1
  spline S585 degree 3 poles (-44.2093, -125.5015) (-44.7896, -124.3091) (-45.3383, -122.8951) (-45.4861, -122.2304) knots 0 0 0 0 1 1 1 1
  spline S586 degree 3 poles (-45.4861, -122.2304) (-45.676, -121.3862) (-45.8237, -120.9008) (-45.8343, -121.1013) knots 0 0 0 0 1 1 1 1
  spline S587 degree 3 poles (-45.8343, -121.1013) (-45.8765, -122.2726) (-44.2831, -126.1346) (-43.0802, -127.7385) knots 0 0 0 0 1 1 1 1
  spline S588 degree 3 poles (-43.0802, -127.7385) (-42.827, -128.0762) (-42.5737, -128.4455) (-42.521, -128.551) knots 0 0 0 0 1 1 1 1
  spline S589 degree 3 poles (-42.521, -128.551) (-42.4576, -128.6671) (-42.12, -128.9837) (-41.7507, -129.2686) knots 0 0 0 0 1 1 1 1
  spline S590 degree 3 poles (-41.7507, -129.2686) (-41.3813, -129.5429) (-41.1386, -129.7751) (-41.2019, -129.7751) knots 0 0 0 0 1 1 1 1
  spline S591 degree 3 poles (-41.2019, -129.7751) (-41.2653, -129.7751) (-41.6873, -129.6273) (-42.1305, -129.4374) knots 0 0 0 0 1 1 1 1
  spline S592 degree 3 poles (-42.1305, -129.4374) (-43.1857, -129.0048) (-43.7661, -128.4244) (-44.3465, -127.2426) knots 0 0 0 0 1 1 1 1
  spline S593 degree 3 poles (-44.3465, -127.2426) (-44.5891, -126.7466) (-44.7896, -126.409) (-44.7896, -126.4828) knots 0 0 0 0 1 1 1 1
  spline S594 degree 3 poles (-44.7896, -126.4828) (-44.7896, -126.5673) (-44.5575, -127.116) (-44.2726, -127.6963) knots 0 0 0 0 1 1 1 1
  spline S595 degree 3 poles (-44.2726, -127.6963) (-43.9877, -128.2872) (-43.6817, -128.9415) (-43.5973, -129.1525) knots 0 0 0 0 1 1 1 1
  spline S596 degree 3 poles (-43.5973, -129.1525) (-43.439, -129.5218) (-43.4495, -129.5324) (-43.6922, -129.4796) knots 0 0 0 0 1 1 1 1
  spline S597 degree 3 poles (-43.6922, -129.4796) (-43.84, -129.4585) (-43.9771, -129.3952) (-44.0088, -129.3424) knots 0 0 0 0 1 1 1 1
  spline S598 degree 3 poles (-44.0088, -129.3424) (-44.0404, -129.2897) (-44.1671, -129.2475) (-44.3042, -129.2475) knots 0 0 0 0 1 1 1 1
  spline S599 degree 3 poles (-44.3042, -129.2475) (-44.7052, -129.2475) (-45.8132, -128.6354) (-46.4252, -128.0656) knots 0 0 0 0 1 1 1 1
  spline S600 degree 3 poles (-46.4252, -128.0656) (-47.1005, -127.4431) (-47.2272, -127.116) (-47.2272, -125.8497) knots 0 0 0 0 1 1 1 1
  spline S601 degree 3 poles (-47.2272, -125.8497) (-47.2272, -125.0794) (-47.1638, -124.8156) (-46.7312, -123.6021) knots 0 0 0 0 1 1 1 1
  spline S602 degree 3 poles (-46.7312, -123.6021) (-46.3302, -122.4836) (-46.0137, -121.4706) (-45.9609, -121.1752) knots 0 0 0 0 1 1 1 1
  spline S603 degree 3 poles (-45.9609, -121.1752) (-45.9504, -121.1435) (-45.9504, -120.9325) (-45.9504, -120.7003) knots 0 0 0 0 1 1 1 1
  line L108 (-45.9504, -120.7003) -> (-45.9504, -120.2888)
  line L109 (-45.9504, -120.2888) -> (-45.4966, -120.4893)
  spline S604 degree 3 poles (-45.4966, -120.4893) (-45.2539, -120.6054) (-44.8952, -120.7003) (-44.6947, -120.7003) knots 0 0 0 0 1 1 1 1
  line L110 (-44.6947, -120.7003) -> (-44.3253, -120.7003)
  line L111 (-44.3253, -120.7003) -> (-44.5891, -120.4049)
  spline S605 degree 3 poles (-44.5891, -120.4049) (-44.7263, -120.2466) (-44.9585, -119.9617) (-45.0851, -119.7823) knots 0 0 0 0 1 1 1 1
  line L112 (-45.0851, -119.7823) -> (-45.3172, -119.4341)
  line L113 (-45.3172, -119.4341) -> (-45.0323, -119.5502)
  spline S606 degree 3 poles (-45.0323, -119.5502) (-44.6103, -119.719) (-43.4495, -119.6768) (-43.1224, -119.4763) knots 0 0 0 0 1 1 1 1
  line L114 (-43.1224, -119.4763) -> (-42.8375, -119.318)
  line L115 (-42.8375, -119.318) -> (-43.1541, -119.3919)
  spline S607 degree 3 poles (-43.1541, -119.3919) (-43.3229, -119.4341) (-43.8189, -119.4657) (-44.2409, -119.4763) knots 0 0 0 0 1 1 1 1
  spline S608 degree 3 poles (-44.2409, -119.4763) (-44.8635, -119.4763) (-45.064, -119.4341) (-45.3172, -119.2441) knots 0 0 0 0 1 1 1 1
  spline S609 degree 3 poles (-45.3172, -119.2441) (-45.4861, -119.1175) (-45.6444, -119.012) (-45.676, -119.012) knots 0 0 0 0 1 1 1 1
  spline S610 degree 3 poles (-45.676, -119.012) (-45.7077, -119.012) (-45.4966, -119.3602) (-45.2223, -119.7717) knots 0 0 0 0 1 1 1 1
  spline S611 degree 3 poles (-45.2223, -119.7717) (-44.9374, -120.1938) (-44.7158, -120.5526) (-44.7369, -120.5631) knots 0 0 0 0 1 1 1 1
  spline S612 degree 3 poles (-44.7369, -120.5631) (-44.8002, -120.6476) (-45.7393, -120.236) (-45.9715, -120.0144) knots 0 0 0 0 1 1 1 1
  spline S613 degree 3 poles (-45.9715, -120.0144) (-46.3408, -119.6768) (-46.4252, -119.6768) (-46.2036, -120.025) knots 0 0 0 0 1 1 1 1
  spline S614 degree 3 poles (-46.2036, -120.025) (-46.0453, -120.2571) (-46.0348, -120.3732) (-46.1614, -121.0485) knots 0 0 0 0 1 1 1 1
  spline S615 degree 3 poles (-46.1614, -121.0485) (-46.2353, -121.4706) (-46.4569, -122.2831) (-46.6573, -122.8635) knots 0 0 0 0 1 1 1 1
  spline S616 degree 3 poles (-46.6573, -122.8635) (-46.8473, -123.4439) (-47.1111, -124.2247) (-47.2166, -124.6046) knots 0 0 0 0 1 1 1 1
  spline S617 degree 3 poles (-47.2166, -124.6046) (-47.4487, -125.3538) (-47.491, -126.4301) (-47.3116, -126.8944) knots 0 0 0 0 1 1 1 1
  spline S618 degree 3 poles (-47.3116, -126.8944) (-47.0372, -127.6225) (-47.6914, -126.4828) (-48.1452, -125.4487) knots 0 0 0 0 1 1 1 1
  spline S619 degree 3 poles (-48.1452, -125.4487) (-48.4195, -124.8367) (-48.6728, -123.8237) (-48.7044, -123.2645) knots 0 0 0 0 1 1 1 1
  spline S620 degree 3 poles (-48.7044, -123.2645) (-48.7255, -123.0218) (-48.7678, -122.8424) (-48.8205, -122.874) knots 0 0 0 0 1 1 1 1
  spline S621 degree 3 poles (-48.8205, -122.874) (-49.0843, -123.0429) (-48.6306, -124.784) (-47.9552, -126.1452) knots 0 0 0 0 1 1 1 1
  spline S622 degree 3 poles (-47.9552, -126.1452) (-47.1638, -127.7702) (-46.0559, -128.857) (-44.8107, -129.258) knots 0 0 0 0 1 1 1 1
  spline S623 degree 3 poles (-44.8107, -129.258) (-44.3253, -129.4057) (-44.2726, -129.448) (-44.5258, -129.448) knots 0 0 0 0 1 1 1 1
  spline S624 degree 3 poles (-44.5258, -129.448) (-45.3594, -129.4585) (-46.9634, -128.6777) (-47.5754, -127.9601) knots 0 0 0 0 1 1 1 1
  spline S625 degree 3 poles (-47.5754, -127.9601) (-47.7864, -127.7174) (-47.9552, -127.5802) (-47.9552, -127.6436) knots 0 0 0 0 1 1 1 1
  spline S626 degree 3 poles (-47.9552, -127.6436) (-47.9552, -127.7174) (-47.6492, -128.0762) (-47.2799, -128.435) knots 0 0 0 0 1 1 1 1
  spline S627 degree 3 poles (-47.2799, -128.435) (-46.6679, -129.0259) (-46.383, -129.3952) (-45.7077, -130.4398) knots 0 0 0 0 1 1 1 1
  spline S628 degree 3 poles (-45.7077, -130.4398) (-45.4228, -130.8725) (-45.6338, -130.7881) (-46.3197, -130.176) knots 0 0 0 0 1 1 1 1
  spline S629 degree 3 poles (-46.3197, -130.176) (-46.7945, -129.754) (-46.8895, -129.7012) (-46.7207, -129.9439) knots 0 0 0 0 1 1 1 1
  spline S630 degree 3 poles (-46.7207, -129.9439) (-46.3408, -130.4821) (-45.2645, -131.1468) (-44.6525, -131.2207) knots 0 0 0 0 1 1 1 1
  line L116 (-44.6525, -131.2207) -> (-44.1249, -131.284)
  line L117 (-44.1249, -131.284) -> (-44.5364, -131.5056)
  spline S631 degree 3 poles (-44.5364, -131.5056) (-44.8635, -131.6744) (-45.1379, -131.7272) (-45.8448, -131.7272) knots 0 0 0 0 1 1 1 1
  spline S632 degree 3 poles (-45.8448, -131.7272) (-46.9739, -131.7166) (-47.5332, -131.4739) (-48.4512, -130.5559) knots 0 0 0 0 1 1 1 1
  spline S633 degree 3 poles (-48.4512, -130.5559) (-49.021, -129.9861) (-49.116, -129.8489) (-49.1265, -129.4902) knots 0 0 0 0 1 1 1 1
  line L118 (-49.1265, -129.4902) -> (-49.1476, -129.0892)
  line L119 (-49.1476, -129.0892) -> (-49.2215, -129.4585)
  spline S634 degree 3 poles (-49.2215, -129.4585) (-49.3059, -129.8806) (-49.2743, -131.2735) (-49.1793, -131.6744) knots 0 0 0 0 1 1 1 1
  spline S635 degree 3 poles (-49.1793, -131.6744) (-49.021, -132.297) (-49.4431, -131.2207) (-49.633, -130.4926) knots 0 0 0 0 1 1 1 1
  spline S636 degree 3 poles (-49.633, -130.4926) (-50.0234, -129.0259) (-50.0129, -127.4009) (-49.5803, -125.3538) knots 0 0 0 0 1 1 1 1
  spline S637 degree 3 poles (-49.5803, -125.3538) (-49.5381, -125.1322) (-49.5486, -125.1111) (-49.633, -125.2588) knots 0 0 0 0 1 1 1 1
  spline S638 degree 3 poles (-49.633, -125.2588) (-49.6963, -125.3538) (-49.7913, -125.6809) (-49.8546, -125.9974) knots 0 0 0 0 1 1 1 1